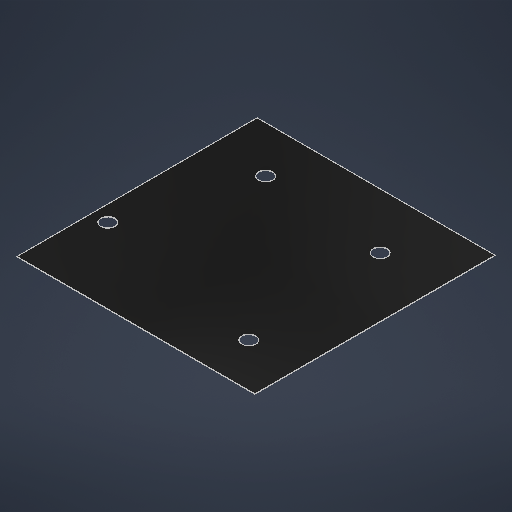
# Autodesk Inventor part: Sensor Placement Film
Saved by Autodesk Inventor 2027 (Build 310192060, 192F)
## iProperties
Created: 2022-02-23
Part Number: Sensor Placement Film
Material: Thermoplastic Resin
Document SubType Name: Modeling
Designer: Caleb
Density: 1.28 g/cm^3
Appearance: Smooth - Black
Author: Caleb
Autodesk Inventor part; units mm, degrees
ref_plane "YZ Plane" through (0, 0, 0) normal (1, 0, 0) x (0, 1, 0)
ref_plane "XZ Plane" through (0, 0, 0) normal (0, 1, 0) x (-1, 0, 0)
ref_plane "XY Plane" through (0, 0, 0) normal (0, 0, 1) x (1, 0, 0)
sketch "Sketch1" plane through (0, 0, 0) normal (0, 1, 0) x (-1, 0, 0)
  line L0 (-21, -21.2) -> (21, -21.2)
  line L1 (21, -21.2) -> (21, 21.2)
  line L2 (21, 21.2) -> (-21, 21.2)
  line L3 (-21, 21.2) -> (-21, -21.2)
  line L4 (-21, -21.2) -> (21, 21.2) construction
  line L5 (21, -21.2) -> (-21, 21.2) construction
  point P0 (0, 0)
  dimension "d0" = 42.4
  dimension "d1" = 42
  constraints: 12 end point, 2 midpoint, 2 parallel, 1 horizontal, 1 perpendicular
  measures "d0" distance of L0.end L1.end
  measures "d1" distance of L1.end L2.end
extrude "Extrusion1" add sketch "Sketch1" along normal blind 0.08
sketch "Sketch2" plane through (0, 0.08, 0) normal (0, 1, 0) x (1, 0, 0)
  circle A0 centre (-11.3636, 13.0568) radius 1.25
  circle A1 centre (10.4908, 11.416) radius 1.25
  circle A2 centre (-18.2, -7.95) radius 1.25
  circle A3 centre (12.2184, -13.4843) radius 1.25
  line L0 (-21, -21.2) -> (21, -21.2) projected
  line L1 (-21, 21.2) -> (-21, -21.2) projected
  point P0 (0, 0)
  dimension "d4" = 2.5
  dimension "d5" = 13.25
  dimension "d6" = 2.8
  constraints: 4 centre point, 3 equal radius
  measures "d4" diameter of A0
  measures "d5" distance from line of A2.centre L0
  measures "d6" distance from line of L1 A2.centre
extrude "Extrusion2" cut sketch "Sketch2" against normal through all
body "Solid1"
